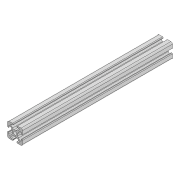
# Autodesk Inventor part: BREEZE-M02
Saved by Autodesk Inventor 2020 (Build 240168000, 168)
## iProperties
Created: 2020-04-12
Part Number: BREEZE-M02
Material: Generic
Document SubType Name: Modeling
Designer: John K
Density: 1 g/cm^3
Appearance: Default
Description: VERTICAL MEMBER
Author: John K
Autodesk Inventor part; units mm, degrees
ref_plane "YZ Plane" through (0, 0, 0) normal (1, 0, 0) x (0, 1, 0)
ref_plane "XZ Plane" through (0, 0, 0) normal (0, 1, 0) x (-1, 0, 0)
ref_plane "XY Plane" through (0, 0, 0) normal (0, 0, 1) x (1, 0, 0)
sketch "Face" plane through (0, 0, 0) normal (0, 0, 1) x (1, 0, 0)
  line L0 (-2.0066, -17.9832) -> (-2.0066, -13.2842)
  line L1 (-0.2032, -12.8016) -> (-0.2032, -14.9098)
  arc A0 (-0.2032, -12.8016) -> (-0.508, -12.4968) centre (-0.508, -12.8016) ccw
  line L2 (-1.2192, -12.4968) -> (-0.508, -12.4968)
  arc A1 (-1.2192, -12.4968) -> (-2.0066, -13.2842) centre (-1.2192, -13.2842) ccw
  arc A2 (4.699, -19.9898) -> (5.4864, -19.2024) centre (4.699, -19.2024) ccw
  arc A3 (-2.0066, -17.9832) -> (0, -19.9898) centre (0, -17.9832) ccw
  arc A4 (-0.2032, -14.9098) -> (1.2277, -15.5025) centre (0.635, -14.9098) ccw
  line L3 (1.2277, -15.5025) -> (3.4825, -13.2477)
  line L4 (4.7355, -14.5007) -> (2.4807, -16.7555)
  arc A5 (2.4807, -16.7555) -> (3.0734, -18.1864) centre (3.0734, -17.3482) ccw
  line L5 (4.699, -19.9898) -> (0, -19.9898)
  line L6 (3.0734, -18.1864) -> (5.1816, -18.1864)
  arc A6 (5.4864, -18.4912) -> (5.1816, -18.1864) centre (5.1816, -18.4912) ccw
  line L7 (5.4864, -18.4912) -> (5.4864, -19.2024)
  line L8 (6.8549, -6.367) -> (9.1217, -6.367)
  arc A7 (4.7355, -5.4891) -> (6.8549, -6.367) centre (6.8549, -3.3698) ccw
  arc A8 (-0.508, -7.493) -> (-0.2032, -7.1882) centre (-0.508, -7.1882) ccw
  circle A9 centre (7.9883, -9.9949) radius 2.1463
  arc A10 (4.3604, -8.8615) -> (3.4825, -6.7421) centre (1.3632, -8.8615) ccw
  line L9 (4.3604, -11.1283) -> (4.3604, -8.8615)
  line L10 (-0.508, -7.493) -> (-1.2192, -7.493)
  arc A11 (16.1798, -5.08) -> (14.7489, -4.4873) centre (15.3416, -5.08) ccw
  line L11 (17.9832, -2.0066) -> (17.9832, -6.7056)
  arc A12 (17.9832, -2.0066) -> (15.9766, 0) centre (15.9766, -2.0066) ccw
  line L12 (14.7489, -4.4873) -> (12.4941, -6.7421)
  arc A13 (13.4959, -3.2343) -> (12.9032, -1.8034) centre (12.9032, -2.6416) ccw
  line L13 (11.2411, -5.4891) -> (13.4959, -3.2343)
  line L14 (11.2776, 0) -> (15.9766, 0)
  line L15 (12.9032, -1.8034) -> (10.795, -1.8034)
  arc A14 (10.4902, -1.4986) -> (10.795, -1.8034) centre (10.795, -1.4986) ccw
  line L16 (10.4902, -1.4986) -> (10.4902, -0.7874)
  arc A15 (11.2776, 0) -> (10.4902, -0.7874) centre (11.2776, -0.7874) ccw
  arc A16 (9.1217, -6.367) -> (11.2411, -5.4891) centre (9.1217, -3.3698) ccw
  line L17 (10.795, -18.1864) -> (12.9032, -18.1864)
  arc A17 (10.4902, -19.2024) -> (11.2776, -19.9898) centre (11.2776, -19.2024) ccw
  line L18 (10.4902, -19.2024) -> (10.4902, -18.4912)
  arc A18 (10.795, -18.1864) -> (10.4902, -18.4912) centre (10.795, -18.4912) ccw
  arc A19 (5.1816, -1.8034) -> (5.4864, -1.4986) centre (5.1816, -1.4986) ccw
  line L19 (5.4864, -0.7874) -> (5.4864, -1.4986)
  line L20 (2.4807, -3.2343) -> (4.7355, -5.4891)
  line L21 (5.1816, -1.8034) -> (3.0734, -1.8034)
  arc A20 (3.0734, -1.8034) -> (2.4807, -3.2343) centre (3.0734, -2.6416) ccw
  line L22 (3.4825, -6.7421) -> (1.2277, -4.4873)
  line L23 (-0.2032, -5.08) -> (-0.2032, -7.1882)
  arc A21 (1.2277, -4.4873) -> (-0.2032, -5.08) centre (0.635, -5.08) ccw
  arc A22 (-2.0066, -6.7056) -> (-1.2192, -7.493) centre (-1.2192, -6.7056) ccw
  line L24 (-2.0066, -6.7056) -> (-2.0066, -2.0066)
  line L25 (0, 0) -> (4.699, 0)
  arc A23 (0, 0) -> (-2.0066, -2.0066) centre (0, -2.0066) ccw
  arc A24 (5.4864, -0.7874) -> (4.699, 0) centre (4.699, -0.7874) ccw
  line L26 (16.1798, -7.1882) -> (16.1798, -5.08)
  arc A25 (17.1958, -7.493) -> (17.9832, -6.7056) centre (17.1958, -6.7056) ccw
  arc A26 (12.9032, -18.1864) -> (13.4959, -16.7555) centre (12.9032, -17.3482) ccw
  line L27 (13.4959, -16.7555) -> (11.2411, -14.5007)
  arc A27 (14.7489, -15.5025) -> (16.1798, -14.9098) centre (15.3416, -14.9098) ccw
  line L28 (12.4941, -13.2477) -> (14.7489, -15.5025)
  line L29 (16.1798, -14.9098) -> (16.1798, -12.8016)
  arc A28 (17.9832, -13.2842) -> (17.1958, -12.4968) centre (17.1958, -13.2842) ccw
  line L30 (17.9832, -13.2842) -> (17.9832, -17.9832)
  arc A29 (15.9766, -19.9898) -> (17.9832, -17.9832) centre (15.9766, -17.9832) ccw
  line L31 (15.9766, -19.9898) -> (11.2776, -19.9898)
  line L32 (17.1958, -7.493) -> (16.4846, -7.493)
  arc A30 (16.1798, -7.1882) -> (16.4846, -7.493) centre (16.4846, -7.1882) ccw
  arc A31 (12.4941, -6.7421) -> (11.6162, -8.8615) centre (14.6134, -8.8615) ccw
  line L33 (11.6162, -8.8615) -> (11.6162, -11.1283)
  arc A32 (11.6162, -11.1283) -> (12.4941, -13.2477) centre (14.6134, -11.1283) ccw
  arc A33 (16.4846, -12.4968) -> (16.1798, -12.8016) centre (16.4846, -12.8016) ccw
  line L34 (16.4846, -12.4968) -> (17.1958, -12.4968)
  arc A34 (3.4825, -13.2477) -> (4.3604, -11.1283) centre (1.3632, -11.1283) ccw
  arc A35 (6.8549, -13.6228) -> (4.7355, -14.5007) centre (6.8549, -16.62) ccw
  line L35 (9.1217, -13.6228) -> (6.8549, -13.6228)
  arc A36 (11.2411, -14.5007) -> (9.1217, -13.6228) centre (9.1217, -16.62) ccw
  point P0 (7.9883, -9.9949)
  point P1 (7.9883, -9.9949)
sketch "Sketch1" plane through (0, 0, 0) normal (0, 0, 1) x (1, 0, 0)
  line L0 (-9.9949, -7.9883) -> (-9.9949, -3.2893)
  line L1 (-8.1915, -2.8067) -> (-8.1915, -4.9149)
  arc A0 (-8.1915, -2.8067) -> (-8.4963, -2.5019) centre (-8.4963, -2.8067) ccw
  line L2 (-9.2075, -2.5019) -> (-8.4963, -2.5019)
  arc A1 (-9.2075, -2.5019) -> (-9.9949, -3.2893) centre (-9.2075, -3.2893) ccw
  arc A2 (-3.2893, -9.9949) -> (-2.5019, -9.2075) centre (-3.2893, -9.2075) ccw
  arc A3 (-9.9949, -7.9883) -> (-7.9883, -9.9949) centre (-7.9883, -7.9883) ccw
  arc A4 (-8.1915, -4.9149) -> (-6.7606, -5.5076) centre (-7.3533, -4.9149) ccw
  line L3 (-6.7606, -5.5076) -> (-4.5058, -3.2528)
  line L4 (-3.2528, -4.5058) -> (-5.5076, -6.7606)
  arc A5 (-5.5076, -6.7606) -> (-4.9149, -8.1915) centre (-4.9149, -7.3533) ccw
  line L5 (-3.2893, -9.9949) -> (-7.9883, -9.9949)
  line L6 (-4.9149, -8.1915) -> (-2.8067, -8.1915)
  arc A6 (-2.5019, -8.4963) -> (-2.8067, -8.1915) centre (-2.8067, -8.4963) ccw
  line L7 (-2.5019, -8.4963) -> (-2.5019, -9.2075)
  line L8 (-1.1334, 3.6279) -> (1.1334, 3.6279)
  arc A7 (-3.2528, 4.5058) -> (-1.1334, 3.6279) centre (-1.1334, 6.6251) ccw
  arc A8 (-8.4963, 2.5019) -> (-8.1915, 2.8067) centre (-8.4963, 2.8067) ccw
  circle A9 centre (0, 0) radius 2.1463
  arc A10 (-3.6279, 1.1334) -> (-4.5058, 3.2528) centre (-6.6251, 1.1334) ccw
  line L9 (-3.6279, -1.1334) -> (-3.6279, 1.1334)
  line L10 (-8.4963, 2.5019) -> (-9.2075, 2.5019)
  arc A11 (8.1915, 4.9149) -> (6.7606, 5.5076) centre (7.3533, 4.9149) ccw
  line L11 (9.9949, 7.9883) -> (9.9949, 3.2893)
  arc A12 (9.9949, 7.9883) -> (7.9883, 9.9949) centre (7.9883, 7.9883) ccw
  line L12 (6.7606, 5.5076) -> (4.5058, 3.2528)
  arc A13 (5.5076, 6.7606) -> (4.9149, 8.1915) centre (4.9149, 7.3533) ccw
  line L13 (3.2528, 4.5058) -> (5.5076, 6.7606)
  line L14 (3.2893, 9.9949) -> (7.9883, 9.9949)
  line L15 (4.9149, 8.1915) -> (2.8067, 8.1915)
  arc A14 (2.5019, 8.4963) -> (2.8067, 8.1915) centre (2.8067, 8.4963) ccw
  line L16 (2.5019, 8.4963) -> (2.5019, 9.2075)
  arc A15 (3.2893, 9.9949) -> (2.5019, 9.2075) centre (3.2893, 9.2075) ccw
  arc A16 (1.1334, 3.6279) -> (3.2528, 4.5058) centre (1.1334, 6.6251) ccw
  line L17 (2.8067, -8.1915) -> (4.9149, -8.1915)
  arc A17 (2.5019, -9.2075) -> (3.2893, -9.9949) centre (3.2893, -9.2075) ccw
  line L18 (2.5019, -9.2075) -> (2.5019, -8.4963)
  arc A18 (2.8067, -8.1915) -> (2.5019, -8.4963) centre (2.8067, -8.4963) ccw
  arc A19 (-2.8067, 8.1915) -> (-2.5019, 8.4963) centre (-2.8067, 8.4963) ccw
  line L19 (-2.5019, 9.2075) -> (-2.5019, 8.4963)
  line L20 (-5.5076, 6.7606) -> (-3.2528, 4.5058)
  line L21 (-2.8067, 8.1915) -> (-4.9149, 8.1915)
  arc A20 (-4.9149, 8.1915) -> (-5.5076, 6.7606) centre (-4.9149, 7.3533) ccw
  line L22 (-4.5058, 3.2528) -> (-6.7606, 5.5076)
  line L23 (-8.1915, 4.9149) -> (-8.1915, 2.8067)
  arc A21 (-6.7606, 5.5076) -> (-8.1915, 4.9149) centre (-7.3533, 4.9149) ccw
  arc A22 (-9.9949, 3.2893) -> (-9.2075, 2.5019) centre (-9.2075, 3.2893) ccw
  line L24 (-9.9949, 3.2893) -> (-9.9949, 7.9883)
  line L25 (-7.9883, 9.9949) -> (-3.2893, 9.9949)
  arc A23 (-7.9883, 9.9949) -> (-9.9949, 7.9883) centre (-7.9883, 7.9883) ccw
  arc A24 (-2.5019, 9.2075) -> (-3.2893, 9.9949) centre (-3.2893, 9.2075) ccw
  line L26 (8.1915, 2.8067) -> (8.1915, 4.9149)
  arc A25 (9.2075, 2.5019) -> (9.9949, 3.2893) centre (9.2075, 3.2893) ccw
  arc A26 (4.9149, -8.1915) -> (5.5076, -6.7606) centre (4.9149, -7.3533) ccw
  line L27 (5.5076, -6.7606) -> (3.2528, -4.5058)
  arc A27 (6.7606, -5.5076) -> (8.1915, -4.9149) centre (7.3533, -4.9149) ccw
  line L28 (4.5058, -3.2528) -> (6.7606, -5.5076)
  line L29 (8.1915, -4.9149) -> (8.1915, -2.8067)
  arc A28 (9.9949, -3.2893) -> (9.2075, -2.5019) centre (9.2075, -3.2893) ccw
  line L30 (9.9949, -3.2893) -> (9.9949, -7.9883)
  arc A29 (7.9883, -9.9949) -> (9.9949, -7.9883) centre (7.9883, -7.9883) ccw
  line L31 (7.9883, -9.9949) -> (3.2893, -9.9949)
  line L32 (9.2075, 2.5019) -> (8.4963, 2.5019)
  arc A30 (8.1915, 2.8067) -> (8.4963, 2.5019) centre (8.4963, 2.8067) ccw
  arc A31 (4.5058, 3.2528) -> (3.6279, 1.1334) centre (6.6251, 1.1334) ccw
  line L33 (3.6279, 1.1334) -> (3.6279, -1.1334)
  arc A32 (3.6279, -1.1334) -> (4.5058, -3.2528) centre (6.6251, -1.1334) ccw
  arc A33 (8.4963, -2.5019) -> (8.1915, -2.8067) centre (8.4963, -2.8067) ccw
  line L34 (8.4963, -2.5019) -> (9.2075, -2.5019)
  arc A34 (-4.5058, -3.2528) -> (-3.6279, -1.1334) centre (-6.6251, -1.1334) ccw
  arc A35 (-1.1334, -3.6279) -> (-3.2528, -4.5058) centre (-1.1334, -6.6251) ccw
  line L35 (1.1334, -3.6279) -> (-1.1334, -3.6279)
  arc A36 (3.2528, -4.5058) -> (1.1334, -3.6279) centre (1.1334, -6.6251) ccw
  point P0 (0, 0)
  constraints: 1 other
extrude "Extrusion1" add sketch "Sketch1" along normal mid plane 200.5
body "Solid1"
